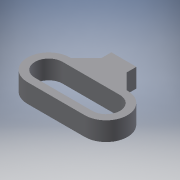
# Autodesk Inventor part: yoke
Saved by Autodesk Inventor 2017 (Build 210142000, 142)
## iProperties
Created: 2018-01-02
Part Number: yoke
Material: Generic
Document SubType Name: Modeling
Designer: RLanting
Density: 1 g/cm^3
Appearance: Default
Author: RLanting
Autodesk Inventor part; units mm, degrees
ref_plane "YZ Plane" through (0, 0, 0) normal (1, 0, 0) x (0, 1, 0)
ref_plane "XZ Plane" through (0, 0, 0) normal (0, 1, 0) x (-1, 0, 0)
ref_plane "XY Plane" through (0, 0, 0) normal (0, 0, 1) x (1, 0, 0)
sketch "Sketch1" plane through (0, 0, 0) normal (0, 0, 1) x (1, 0, 0)
  line L0 (22.86, 0) -> (-22.86, 0) construction
  line L1 (22.86, 11) -> (-22.86, 11)
  line L2 (-22.86, -11) -> (22.86, -11)
  arc A0 (22.86, -11) -> (22.86, 11) centre (22.86, 0) ccw
  arc A1 (-22.86, 11) -> (-22.86, -11) centre (-22.86, 0) ccw
  line L3 (22.86, 0) -> (-22.86, 0) construction
  line L4 (22.86, 17) -> (-22.86, 17)
  line L5 (-22.86, -17) -> (22.86, -17)
  arc A2 (22.86, -17) -> (22.86, 17) centre (22.86, 0) ccw
  arc A3 (-22.86, 17) -> (-22.86, -17) centre (-22.86, 0) ccw
  line L6 (-10, 17) -> (10, 17)
  line L7 (10, 17) -> (10, 37)
  line L8 (10, 37) -> (-10, 37)
  line L9 (-10, 37) -> (-10, 17)
  point P0 (0, 0)
  point P1 (0, 17)
  dimension "d0" = 22
  dimension "d1" = 6
  dimension "d2" = 45.72
  dimension "d3" = 20
  dimension "d4" = 20
  constraints: 24 end point, 8 point on circle, 8 tangent, 5 equal length, 4 centre point, 4 midpoint, 2 horizontal, 1 perpendicular, 1 point on line
  measures "d0" distance between parallel lines of L2 L1
  measures "d1" distance between parallel lines of L1 L4
  measures "d2" distance of L0.start L0.end
  measures "d3" distance of L7.end L8.end
  measures "d4" distance of L8.end L6.start
extrude "Extrusion1" add sketch "Sketch1" along normal blind 15
sketch "Sketch2" plane through (-10, 37, 0) normal (0, 1, 0) x (1, 0, 0)
  line L0 (-12.86, -15) -> (32.86, -15) construction
  line L1 (10, -15) -> (10, 0) construction
  circle A0 centre (10, -7.5) radius 3.5
  dimension "d7" = 7
  constraints: 2 end point, 2 midpoint, 1 centre point, 1 vertical
  measures "d7" diameter of A0
extrude "Extrusion2" cut sketch "Sketch2" against normal blind 15
chamfer "Chamfer1" distance 12.25 angle 45 2 edges at (10, 17, 7.5) (-10, 17, 7.5)
body "Solid1"
